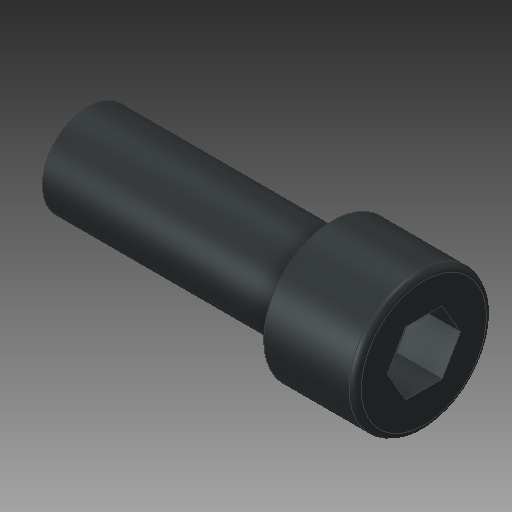
# Autodesk Inventor part: M3
Saved by Autodesk Inventor 2019 (Build 230136000, 136)
## iProperties
Created: 2020-02-22
Part Number: M3
Material: Iron, Cast
Document SubType Name: Modeling
Designer: Elías Sánchez
Density: 7.15 g/cm^3
Appearance: Iron Gray
Description: La Casa del Tormillo
Author: Elías Sánchez
Revision Number: IR
Autodesk Inventor part; units mm, degrees
ref_plane "YZ Plane" through (0, 0, 0) normal (1, 0, 0) x (0, 1, 0)
ref_plane "XZ Plane" through (0, 0, 0) normal (0, 1, 0) x (-1, 0, 0)
sketch "Sketch1" plane through (0, 0, 0) normal (1, 0, 0) x (0, 1, 0)
  circle A0 centre (0, 0) radius 1.5
  dimension "d0" = 3
  constraints: 1 centre point, 1 coincident
  measures "d0" diameter of A0
extrude "Extrusion1" add sketch "Sketch1" along normal blind 8
sketch "Sketch2" plane through (8, 0, 0) normal (1, 0, 0) x (0, 0, -1)
  circle A0 centre (0, 0) radius 2.25
  dimension "d3" = 4.5
  constraints: 1 centre point, 1 coincident
  measures "d3" diameter of A0
extrude "Extrusion2" add sketch "Sketch2" along normal blind 3
ref_plane "Work Plane1" through (13.5, 0, 0) normal (1, 0, 0) x (0, 0, -1)
fillet "Fillet2" radius 0.2 1 edges at (11, 0, 2.25)
sketch "Sketch4" plane through (11, 0, 0) normal (1, 0, 0) x (0, 0, -1)
  line L0 (1.2, 0) -> (0.6, -1.0392)
  line L1 (0.6, -1.0392) -> (-0.6, -1.0392)
  line L2 (-0.6, -1.0392) -> (-1.2, 0)
  line L3 (-1.2, 0) -> (-0.6, 1.0392)
  line L4 (-0.6, 1.0392) -> (0.6, 1.0392)
  line L5 (0.6, 1.0392) -> (1.2, 0)
  point P0 (0, 0)
  point P1 (0, 0)
  dimension "d14" = 2.4
  dimension "d15" = 1.0392
  constraints: 12 end point, 1 coincident, 13 other
  measures "d14" distance of L2.end L0.start
  measures "d15" vertical distance of L4.end L0.start
extrude "Extrusion4" cut sketch "Sketch4" against normal blind 1.5
body "Solid1"
